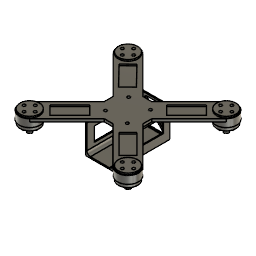
droneframev3 (Autodesk Fusion 360 archive; units mm, degrees)
design "droneTestv2"
part number: 2026-03-09-17-57-18-484
Autodesk Fusion 360 part; units mm, degrees
sketch "Sketch1" plane through (0, 0, 0) normal (0, 0, 1) x (1, 0, 0)
  line L0 (5.1145, 0) -> (50, 0)
  line L1 (55, -5) -> (55, -50)
  line L2 (50, -55) -> (5, -55)
  line L3 (0, -50) -> (0, -5.1145)
  circle A0 centre (12, -11) radius 2
  circle A1 centre (43, -11) radius 2
  circle A2 centre (12, -44) radius 2
  circle A3 centre (43, -44) radius 2
  line L4 (0, -5.1145) -> (0, 0)
  line L5 (0, 0) -> (5.1145, 0)
  line L6 (50, 0) -> (55, 0)
  line L7 (55, 0) -> (55, -5)
  line L8 (50, -55) -> (55, -55)
  line L9 (55, -55) -> (55, -50)
  line L10 (0, -50) -> (0, -55)
  line L11 (0, -55) -> (5, -55)
  line L12 (0, -21.2132) -> (21.2132, 0)
  line L13 (21.2132, 0) -> (-31.8198, 53.033)
  line L14 (-31.8198, 53.033) -> (-53.033, 31.8198)
  line L15 (-53.033, 31.8198) -> (0, -21.2132)
  line L16 (21.2132, -55) -> (0, -33.7868)
  line L17 (0, -33.7868) -> (-53.033, -86.8198)
  line L18 (-53.033, -86.8198) -> (-31.8198, -108.033)
  line L19 (-31.8198, -108.033) -> (21.2132, -55)
  line L20 (33.7868, -55) -> (55, -33.7868)
  line L21 (55, -33.7868) -> (108.033, -86.8198)
  line L22 (108.033, -86.8198) -> (86.8198, -108.033)
  line L23 (86.8198, -108.033) -> (33.7868, -55)
  line L24 (33.7868, 0) -> (55, -21.2132)
  line L25 (55, -21.2132) -> (108.033, 31.8198)
  line L26 (108.033, 31.8198) -> (86.8198, 53.033)
  line L27 (86.8198, 53.033) -> (33.7868, 0)
  circle A4 centre (-40, -95) radius 64.77
  circle A5 centre (95, -95) radius 64.77
  circle A6 centre (-40, 40) radius 64.77
  circle A7 centre (95, 40) radius 64.77
  circle A8 centre (97.4264, -97.4264) radius 8
  circle A9 centre (97.4264, -89.4264) radius 2
  circle A10 centre (105.4264, -97.4264) radius 2
  circle A11 centre (97.4264, -105.4264) radius 2
  circle A12 centre (89.4264, -97.4264) radius 2
  circle A13 centre (97.4264, -97.4264) radius 13.75
  circle A14 centre (97.4264, -97.4264) radius 15
  circle A15 centre (-42.4264, -97.4264) radius 8
  circle A16 centre (-42.4264, -105.4264) radius 2
  circle A17 centre (-50.4264, -97.4264) radius 2
  circle A18 centre (-42.4264, -89.4264) radius 2
  circle A19 centre (-34.4264, -97.4264) radius 2
  circle A20 centre (-42.4264, -97.4264) radius 13.75
  circle A21 centre (-42.4264, -97.4264) radius 15
  circle A22 centre (-42.4264, 42.4264) radius 8
  circle A23 centre (-50.4264, 42.4264) radius 2
  circle A24 centre (-42.4264, 50.4264) radius 2
  circle A25 centre (-34.4264, 42.4264) radius 2
  circle A26 centre (-42.4264, 34.4264) radius 2
  circle A27 centre (-42.4264, 42.4264) radius 15
  circle A28 centre (-42.4264, 42.4264) radius 13.75
  circle A29 centre (97.4264, 42.4264) radius 15
  circle A30 centre (97.4264, 42.4264) radius 13.75
  circle A31 centre (97.4264, 42.4264) radius 8
  circle A32 centre (97.4264, 50.4264) radius 2
  circle A33 centre (105.4264, 42.4264) radius 2
  circle A34 centre (97.4264, 34.4264) radius 2
  circle A35 centre (89.4264, 42.4264) radius 2
  circle A36 centre (97.4264, -105.4264) radius 3
  circle A37 centre (89.4264, -97.4264) radius 3
  circle A38 centre (97.4264, -89.4264) radius 3
  circle A39 centre (105.4264, -97.4264) radius 3
  circle A40 centre (105.4264, 42.4264) radius 3
  circle A41 centre (97.4264, 50.4264) radius 3
  circle A42 centre (89.4264, 42.4264) radius 3
  circle A43 centre (97.4264, 34.4264) radius 3
  circle A44 centre (-34.4264, 42.4264) radius 3
  circle A45 centre (-42.4264, 50.4264) radius 3
  circle A46 centre (-50.4264, 42.4264) radius 3
  circle A47 centre (-42.4264, 34.4264) radius 3
  circle A48 centre (-42.4264, -89.4264) radius 3
  circle A49 centre (-50.4264, -97.4264) radius 3
  circle A50 centre (-34.4264, -97.4264) radius 3
  circle A51 centre (-42.4264, -105.4264) radius 3
  point P0 (55, 0)
  point P1 (0, -55)
  dimension "d1" = 55
  dimension "d2" = 55
  dimension "d7" = 4
  dimension "d8" = 12
  dimension "d9" = 11
  dimension "d11" = 4
  dimension "d12" = 12
  dimension "d13" = 11
  dimension "d14" = 4
  dimension "d15" = 11
  dimension "d16" = 12
  dimension "d17" = 4
  dimension "d18" = 12
  dimension "d19" = 11
  dimension "d22" = 75
  dimension "d23" = 30
  dimension "d24" = 75
  dimension "d25" = 30
  dimension "d26" = 75
  dimension "d27" = 30
  dimension "d28" = 75
  dimension "d29" = 30
  dimension "d31" = 129.54
  dimension "d32" = 129.54
  dimension "d33" = 129.54
  dimension "d34" = 129.54
  dimension "d49" = 16
  dimension "d52" = 4
  dimension "d53" = 4
  dimension "d54" = 4
  dimension "d55" = 4
  dimension "d56" = 27.5
  dimension "d57" = 16
  dimension "d58" = 4
  dimension "d59" = 4
  dimension "d60" = 4
  dimension "d61" = 4
  dimension "d62" = 27.5
  dimension "d63" = 30
  dimension "d64" = 16
  dimension "d65" = 4
  dimension "d66" = 4
  dimension "d67" = 4
  dimension "d68" = 4
  dimension "d69" = 30
  dimension "d70" = 27.5
  dimension "d71" = 30
  dimension "d72" = 27.5
  dimension "d73" = 16
  dimension "d74" = 4
  dimension "d75" = 4
  dimension "d76" = 4
  dimension "d77" = 4
  dimension "d169" = 6
  dimension "d170" = 6
  dimension "d171" = 6
  dimension "d172" = 6
  dimension "d191" = 6
  dimension "d192" = 6
  dimension "d193" = 6
  dimension "d194" = 6
  dimension "d195" = 6
  dimension "d196" = 6
  dimension "d197" = 6
  dimension "d198" = 6
  dimension "d199" = 6
  dimension "d200" = 6
  dimension "d201" = 6
  dimension "d202" = 6
  constraint horizontal L0
  constraint vertical L1
  constraint horizontal L2
  constraint vertical L3
  constraint coincident L4.end L5.start
  constraint coincident L4.end L0
  constraint coincident L4.end L3
  constraint coincident P0 L1
  constraint coincident P0 L0
  constraint coincident P1 L2
  constraint coincident P1 L3
  constraint coincident P0 L6.end
  constraint parallel L2 L8
  constraint coincident P1 L10.end
  constraint perpendicular L12 L13
  constraint parallel L12 L14
  constraint parallel L13 L15
  constraint coincident L0 L12.end
  constraint coincident L3 L12.start
  constraint perpendicular L16 L17
  constraint parallel L16 L18
  constraint parallel L17 L19
  constraint coincident L3 L16.end
  constraint coincident L2 L16.start
  constraint perpendicular L20 L21
  constraint parallel L20 L22
  constraint parallel L21 L23
  constraint coincident L1 L20.end
  constraint coincident L2 L20.start
  constraint perpendicular L24 L25
  constraint parallel L24 L26
  constraint parallel L25 L27
  constraint coincident L1 L24.end
  constraint coincident L0 L24.start
  constraint midpoint L22 A8.centre
  constraint coincident A8 A9.centre
  constraint coincident A8 A10.centre
  constraint coincident A8 A11.centre
  constraint coincident A8 A12.centre
  constraint concentric A8 A13
  constraint concentric A8 A14
  constraint coincident L22.end A14
  constraint midpoint L18 A15.centre
  constraint coincident A15 A16.centre
  constraint coincident A15 A17.centre
  constraint coincident A15 A18.centre
  constraint coincident A15 A19.centre
  constraint concentric A15 A20
  constraint concentric A20 A21
  constraint midpoint L14 A22.centre
  constraint coincident A22 A23.centre
  constraint coincident A22 A24.centre
  constraint coincident A22 A25.centre
  constraint coincident A22 A26.centre
  constraint concentric A22 A27
  constraint concentric A27 A28
  constraint midpoint L26 A29.centre
  constraint concentric A29 A30
  constraint concentric A30 A31
  constraint coincident A31 A32.centre
  constraint coincident A31 A33.centre
  constraint coincident A31 A34.centre
  constraint coincident A31 A35.centre
  constraint concentric A11 A36
  constraint concentric A12 A37
  constraint concentric A9 A38
  constraint concentric A10 A39
  constraint concentric A33 A40
  constraint concentric A32 A41
  constraint concentric A35 A42
  constraint concentric A34 A43
  constraint concentric A25 A44
  constraint concentric A24 A45
  constraint concentric A23 A46
  constraint concentric A26 A47
  constraint concentric A18 A48
  constraint concentric A17 A49
  constraint concentric A19 A50
  constraint concentric A16 A51
  measures "d1" distance of L4.end P0
  measures "d2" distance of L4.end L10.end
  measures "d7" diameter of A0
  measures "d8" distance of L3 A0.centre
  measures "d9" distance of L0 A0.centre
  measures "d11" diameter of A1
  measures "d12" distance of L1 A1.centre
  measures "d13" distance of L0 A1.centre
  measures "d14" diameter of A2
  measures "d15" distance of L2 A2.centre
  measures "d16" distance of L3 A2.centre
  measures "d17" diameter of A3
  measures "d18" distance of L1 A3.centre
  measures "d19" distance of L2 A3.centre
  measures "d22" distance of L12.start L14.end
  measures "d23" distance of L13 L15
  measures "d24" distance of L16.start L18.end
  measures "d25" distance of L17 L19
  measures "d26" distance of L20.start L22.end
  measures "d27" distance of L21 L23
  measures "d28" distance of L24.start L26.end
  measures "d29" distance of L25 L27
  measures "d31" diameter of A4
  measures "d32" diameter of A5
  measures "d33" diameter of A6
  measures "d34" diameter of A7
  measures "d49" diameter of A8
  measures "d52" diameter of A9
  measures "d53" diameter of A10
  measures "d54" diameter of A11
  measures "d55" diameter of A12
  measures "d56" diameter of A13
  measures "d57" diameter of A15
  measures "d58" diameter of A16
  measures "d59" diameter of A17
  measures "d60" diameter of A18
  measures "d61" diameter of A19
  measures "d62" diameter of A20
  measures "d63" diameter of A21
  measures "d64" diameter of A22
  measures "d65" diameter of A23
  measures "d66" diameter of A24
  measures "d67" diameter of A25
  measures "d68" diameter of A26
  measures "d69" diameter of A27
  measures "d70" diameter of A28
  measures "d71" diameter of A29
  measures "d72" diameter of A30
  measures "d73" diameter of A31
  measures "d74" diameter of A32
  measures "d75" diameter of A33
  measures "d76" diameter of A34
  measures "d77" diameter of A35
  measures "d169" diameter of A36
  measures "d170" diameter of A37
  measures "d171" diameter of A38
  measures "d172" diameter of A39
  measures "d191" diameter of A40
  measures "d192" diameter of A41
  measures "d193" diameter of A42
  measures "d194" diameter of A43
  measures "d195" diameter of A44
  measures "d196" diameter of A45
  measures "d197" diameter of A46
  measures "d198" diameter of A47
  measures "d199" diameter of A48
  measures "d200" diameter of A49
  measures "d201" diameter of A50
  measures "d202" diameter of A51
extrude "Extrude1" add sketch "Sketch1" along normal blind 3 contours L0 L3 A0 L12 A6 | L0 L1 L2 L3 A0 A1 A2 A3 L12 L16 L20 L24 | L0 L13 A6 | L0 L27 A7 | L0 L1 A1 L24 A7 | L0 L3 L4 L5 A6 | L0 L3 L4 L5 L13 L15 A6 A27 | L0 L1 L6 L7 L25 L27 A7 A29 | L0 L1 L6 L7 A7 | L3 L15 A6 | L14 A27 A28 | L14 A27 A28 | L1 L25 A7 | L26 A29 A30 | L26 A29 A30 | L14 A22 A28 A44 A47 | L14 A22 A28 A45 A46 | L26 A30 A31 A40 A41 | L26 A30 A31 A42 A43 | L2 L3 A2 L16 A4 | L3 L17 A4 | L14 A22 A44 A47 | L14 A22 A45 A46 | L1 L21 A5 | L1 L2 A3 L20 A5 | L26 A31 A40 A41 | L26 A31 A42 A43 | L2 L3 L10 L11 A4 | L2 L3 L10 L11 L17 L19 A4 A21 | A22 A25 A44 | A22 A25 A44 | A22 A24 A45 | A22 A24 A45 | L1 L2 L8 L9 L21 L23 A5 A14 | L1 L2 L8 L9 A5 | A31 A32 A41 | A31 A32 A41 | A31 A35 A42 | A31 A35 A42 | L2 L19 A4 | L18 A20 A21 | L18 A20 A21 | A22 A23 A46 | A22 A23 A46 | A22 A26 A47 | A22 A26 A47 | L2 L23 A5 | L22 A13 A14 | L22 A13 A14 | A31 A34 A43 | A31 A34 A43 | A31 A33 A40 | A31 A33 A40 | L18 A15 A20 A48 A50 | L18 A15 A20 A49 A51 | L22 A8 A13 A36 A39 | L22 A8 A13 A37 A38 | L18 A15 A48 A50 | L18 A15 A49 A51 | L22 A8 A36 A39 | L22 A8 A37 A38 | A15 A18 A48 | A15 A18 A48 | A15 A17 A49 | A15 A17 A49 | A8 A10 A39 | A8 A10 A39 | A8 A9 A38 | A8 A9 A38 | A15 A16 A51 | A15 A16 A51 | A15 A19 A50 | A15 A19 A50 | A8 A12 A37 | A8 A12 A37 | A8 A11 A36 | A8 A11 A36 makes body 1
extrude "Extrude2" add 1 faces at (-8.062, 10.5564, 3) along direction (0, 0, 1) blind 1 on bodies 1 bodies 1
extrude "Extrude3" cut sketch "Sketch1" along normal blind 10 contours L14 A22 A28 A44 A47 | L14 A22 A28 A45 A46 | L14 A22 A44 A47 | L14 A22 A45 A46 | A22 A25 A44 | A22 A25 A44 | A22 A24 A45 | A22 A24 A45 | A22 A23 A46 | A22 A23 A46 | A22 A26 A47 | A22 A26 A47 bodies 1
extrude "Extrude4" add sketch "Sketch1" along normal blind 10 contours L14 A22 A28 A44 A47 | L14 A22 A28 A45 A46 | L14 A22 A44 A47 | L14 A22 A45 A46 | A22 A25 A44 | A22 A25 A44 | A22 A24 A45 | A22 A24 A45 | A22 A23 A46 | A22 A23 A46 | A22 A26 A47 | A22 A26 A47 bodies 1
extrude "Extrude5" cut sketch "Sketch1" along normal blind 10 contours L26 A30 A31 A40 A41 | L26 A30 A31 A42 A43 | L26 A31 A40 A41 | L26 A31 A42 A43 | A31 A32 A41 | A31 A32 A41 | A31 A35 A42 | A31 A35 A42 | A31 A34 A43 | A31 A34 A43 | A31 A33 A40 | A31 A33 A40 | L18 A15 A20 A48 A50 | L18 A15 A20 A49 A51 | L22 A8 A13 A36 A39 | L22 A8 A13 A37 A38 | L18 A15 A48 A50 | L18 A15 A49 A51 | L22 A8 A36 A39 | L22 A8 A37 A38 | A15 A18 A48 | A15 A18 A48 | A15 A17 A49 | A15 A17 A49 | A8 A10 A39 | A8 A10 A39 | A8 A9 A38 | A8 A9 A38 | A15 A16 A51 | A15 A16 A51 | A15 A19 A50 | A15 A19 A50 | A8 A12 A37 | A8 A12 A37 | A8 A11 A36 | A8 A11 A36 bodies 1
extrude "Extrude6" add sketch "Sketch1" along normal blind 10 contours L26 A30 A31 A40 A41 | L26 A30 A31 A42 A43 | L26 A31 A40 A41 | L26 A31 A42 A43 | A31 A32 A41 | A31 A32 A41 | A31 A35 A42 | A31 A35 A42 | A31 A34 A43 | A31 A34 A43 | A31 A33 A40 | A31 A33 A40 | L18 A15 A20 A48 A50 | L18 A15 A20 A49 A51 | L22 A8 A13 A36 A39 | L22 A8 A13 A37 A38 | L18 A15 A48 A50 | L18 A15 A49 A51 | L22 A8 A36 A39 | L22 A8 A37 A38 | A15 A18 A48 | A15 A18 A48 | A15 A17 A49 | A15 A17 A49 | A8 A10 A39 | A8 A10 A39 | A8 A9 A38 | A8 A9 A38 | A15 A16 A51 | A15 A16 A51 | A15 A19 A50 | A15 A19 A50 | A8 A12 A37 | A8 A12 A37 | A8 A11 A36 | A8 A11 A36 bodies 1
extrude "Extrude7" cut 4 faces at (97.346, 40.4215, 10) (-42.5068, 44.4313, 10) (-42.346, -95.4215, 10) (97.346, -99.4313, 10) along direction (0, 0, -1) blind 5 on bodies 1 bodies 1
extrude "Extrude8" add 1 faces at (97.346, -99.4313, 5) along direction (0, 0, -1) blind 6 on bodies 1 bodies 1
extrude "Extrude9" add 1 faces at (97.346, -99.4313, -1) along direction (0, 0, 1) blind 2 on bodies 1 bodies 1
extrude "Extrude10" add 1 faces at (97.346, -99.4313, -1) along direction (0, 0, -1) blind 2 on bodies 1 bodies 1
extrude "Extrude11" add sketch "Sketch1" against normal blind 7 contours L22 A8 A36 A39 | L22 A8 A37 A38 | A8 A10 A39 | A8 A9 A38 | A8 A12 A37 | A8 A11 A36 | A8 A10 | A8 A9 | A8 A12 | A8 A11 picked at (104.6818, -99.8582) picked at (99.8582, -90.171) picked at (90.1642, -99.8605) picked at (99.8582, -104.6818) picked at (104.7781, -97.839) picked at (96.813, -90.0523) picked at (90.0523, -96.813) picked at (96.813, -104.8005) bodies 1
extrude "Extrude12" add sketch "Sketch1" against normal blind 5 contours A8 A10 | A8 A9 | A8 A12 | A8 A11 picked at (106.0247, -97.9232) picked at (98.0975, -88.8726) picked at (88.8675, -96.764) picked at (98.0975, -105.9803) bodies 1
extrude "Extrude13" add sketch "Sketch1" against normal blind 3 contours L26 A30 A31 A40 A41 | L26 A30 A31 A42 A43 | A31 A32 A41 | A31 A35 A42 | A31 A34 A43 | A31 A33 A40 picked at (94.9952, 50.4291) picked at (89.4207, 44.8573) picked at (94.9952, 34.4237) picked at (105.428, 39.9955) bodies 1
extrude "Extrude14" add sketch "Sketch1" against normal blind 6 contours A31 A32 | A31 A35 | A31 A34 | A31 A33 picked at (98.0975, 50.9803) picked at (88.8675, 41.764) picked at (98.0975, 33.8726) picked at (106.0247, 41.9296) bodies 1
extrude "Extrude15" add sketch "Sketch1" against normal blind 7 contours L26 A31 A40 A41 | L26 A31 A42 A43 | A31 A32 A41 | A31 A35 A42 | A31 A34 A43 | A31 A33 A40 | A31 A32 | A31 A35 | A31 A34 | A31 A33 picked at (94.9947, 49.6818) picked at (90.1642, 39.9923) picked at (94.9947, 35.171) picked at (104.6818, 44.8582) picked at (98.0399, 49.8005) picked at (90.0523, 41.813) picked at (96.813, 35.0523) picked at (104.7781, 42.0138) bodies 1
extrude "Extrude16" add sketch "Sketch1" against normal blind 3 contours L14 A22 A28 A44 A47 | L14 A22 A28 A45 A46 | A22 A25 A44 | A22 A24 A45 | A22 A23 A46 | A22 A26 A47 picked at (-34.4248, 39.9955) picked at (-44.8576, 50.4291) picked at (-50.4321, 44.8573) picked at (-44.8576, 34.4237) bodies 1
extrude "Extrude17" add sketch "Sketch1" against normal blind 6 contours A22 A25 | A22 A24 | A22 A23 | A22 A26 picked at (-33.8281, 41.9296) picked at (-41.7553, 50.9803) picked at (-50.9853, 43.0888) picked at (-41.7553, 33.8726) bodies 1
extrude "Extrude18" add sketch "Sketch1" against normal blind 7 contours L14 A22 A44 A47 | L14 A22 A45 A46 | A22 A25 A44 | A22 A24 A45 | A22 A23 A46 | A22 A26 A47 | A22 A25 | A22 A24 | A22 A23 | A22 A26 picked at (-35.171, 39.9947) picked at (-44.8582, 49.6818) picked at (-49.6886, 44.8605) picked at (-44.8582, 35.171) picked at (-35.0747, 42.0138) picked at (-43.0399, 49.8005) picked at (-49.8005, 41.813) picked at (-43.0399, 35.0523) bodies 1
extrude "Extrude19" add sketch "Sketch1" against normal blind 3 contours L18 A15 A20 A48 A50 | L18 A15 A20 A49 A51 | A15 A18 A48 | A15 A17 A49 | A15 A16 A51 | A15 A19 A50 picked at (-44.8576, -89.4237) picked at (-50.4321, -94.9956) picked at (-44.8576, -105.4291) picked at (-34.4248, -99.8573) bodies 1
extrude "Extrude20" add sketch "Sketch1" against normal blind 6 contours A15 A18 | A15 A17 | A15 A16 | A15 A19 picked at (-41.7553, -88.8726) picked at (-50.9853, -96.764) picked at (-41.7553, -105.9803) picked at (-33.8281, -96.9296) bodies 1
extrude "Extrude21" add sketch "Sketch1" against normal blind 7 contours L18 A15 A48 A50 | L18 A15 A49 A51 | A15 A18 A48 | A15 A17 A49 | A15 A16 A51 | A15 A19 A50 | A15 A18 | A15 A17 | A15 A16 | A15 A19 picked at (-39.9947, -90.171) picked at (-49.6886, -99.8605) picked at (-44.8582, -104.6818) picked at (-35.171, -94.9947) picked at (-43.0399, -90.0523) picked at (-49.8005, -96.813) picked at (-43.0399, -104.8005) picked at (-35.0747, -97.839) bodies 1
extrude "Extrude22" add sketch "Sketch1" against normal blind 12 contours L22 A8 A13 A36 A39 | L22 A8 A13 A37 A38 | A8 A10 A39 | A8 A9 A38 | A8 A12 A37 | A8 A11 A36 picked at (105.428, -99.8573) picked at (94.9952, -89.4237) picked at (89.4207, -94.9956) picked at (94.9952, -105.4291) bodies 1
extrude "Extrude23" add sketch "Sketch1" against normal blind 7 contours L22 A13 A14 | L22 A13 A14 bodies 1
extrude "Extrude24" add sketch "Sketch1" against normal blind 7 contours L22 A13 A14 | L22 A13 A14 bodies 1
extrude "Extrude25" cut sketch "Sketch1" along normal blind -30 and the other way blind -6 contours A8 A10 A39 | A8 A10 A39 | A8 A10 | A8 A10 bodies 1
extrude "Extrude26" add sketch "Sketch1" along normal blind 5 contours A8 A10 A39 | A8 A10 A39 bodies 1
extrude "Extrude27" add 1 faces at (94.1257, -99.2826, -7) along direction (0, 0, -1) blind 11 on bodies 1 bodies 1
extrude "Extrude28" cut sketch "Sketch1" along normal mid plane 60 contours A8 A9 A38 | A8 A9 A38 | A8 A12 A37 | A8 A12 A37 | A8 A11 A36 | A8 A11 A36 | A8 A9 | A8 A9 | A8 A12 | A8 A12 | A8 A11 | A8 A11 bodies 1
extrude "Extrude29" add sketch "Sketch1" along normal blind 5 contours A8 A9 A38 | A8 A9 A38 | A8 A12 A37 | A8 A12 A37 | A8 A11 A36 | A8 A11 A36 bodies 1
extrude "Extrude30" add sketch "Sketch1" against normal blind 7 contours L26 A29 A30 | L26 A29 A30 bodies 1
extrude "Extrude31" add sketch "Sketch1" against normal blind 12 separate body contours L26 A30 A31 A40 A41 | L26 A30 A31 A42 A43 | A31 A32 A41 | A31 A35 A42 | A31 A34 A43 | A31 A33 A40 picked at (94.9952, 50.4291) picked at (89.4207, 44.8573) picked at (94.9952, 34.4237) picked at (105.428, 39.9955) makes body 2
extrude "Extrude32" add sketch "Sketch1" against normal blind 19 separate body contours L26 A31 A40 A41 | L26 A31 A42 A43 | A31 A32 A41 | A31 A35 A42 | A31 A34 A43 | A31 A33 A40 picked at (94.9947, 49.6818) picked at (90.1642, 39.9923) picked at (94.9947, 35.171) picked at (104.6818, 44.8582) makes body 3
extrude "Extrude33" cut sketch "Sketch1" along normal mid plane 40 contours A31 A32 A41 | A31 A32 A41 | A31 A35 A42 | A31 A35 A42 | A31 A34 A43 | A31 A34 A43 | A31 A33 A40 | A31 A33 A40 | A31 A32 | A31 A32 | A31 A35 | A31 A35 | A31 A34 | A31 A34 | A31 A33 | A31 A33 bodies 1 2 3
extrude "Extrude34" add sketch "Sketch1" along normal blind 5 contours A31 A32 A41 | A31 A32 A41 | A31 A35 A42 | A31 A35 A42 | A31 A34 A43 | A31 A34 A43 | A31 A33 A40 | A31 A33 A40 bodies 1 2 3
extrude "Extrude35" add sketch "Sketch1" against normal blind 19 separate body contours L14 A22 A44 A47 | L14 A22 A45 A46 makes body 4
extrude "Extrude36" add sketch "Sketch1" against normal blind 19 separate body contours L14 A22 A28 A44 A47 | L14 A22 A28 A45 A46 makes body 5
extrude "Extrude37" cut 1 faces at (-47.5438, 51.3129, -19) along direction (0, 0, 1) blind 7 on bodies 5 bodies 5
extrude "Extrude38" add sketch "Sketch1" against normal blind 7 contours L14 A27 A28 | L14 A27 A28 bodies 1 5
extrude "Extrude39" cut sketch "Sketch1" along normal mid plane 40 contours A22 A25 A44 | A22 A25 A44 | A22 A24 A45 | A22 A24 A45 | A22 A23 A46 | A22 A23 A46 | A22 A26 A47 | A22 A26 A47 | A22 A25 | A22 A25 | A22 A24 | A22 A24 | A22 A23 | A22 A23 | A22 A26 | A22 A26 bodies 1
extrude "Extrude40" add sketch "Sketch1" along normal blind 5 contours A22 A25 A44 | A22 A25 A44 | A22 A24 A45 | A22 A24 A45 | A22 A23 A46 | A22 A23 A46 | A22 A26 A47 | A22 A26 A47 bodies 1 4
extrude "Extrude41" add 1 faces at (-32.1932, -103.3174, -3) along direction (0, 0, -1) blind 9 on bodies 1 bodies 1
extrude "Extrude42" add sketch "Sketch1" against normal blind 7 contours L18 A20 A21 | L18 A20 A21 bodies 1
extrude "Extrude43" add 1 faces at (-41.6768, -95.0423, -7) along direction (0, 0, -1) blind 12 on bodies 1 bodies 1
extrude "Extrude44" cut sketch "Sketch1" along normal mid plane 40 contours A15 A18 A48 | A15 A18 A48 | A15 A17 A49 | A15 A17 A49 | A15 A16 A51 | A15 A16 A51 | A15 A19 A50 | A15 A19 A50 | A15 A18 | A15 A18 | A15 A17 | A15 A17 | A15 A16 | A15 A16 | A15 A19 | A15 A19 bodies 1
extrude "Extrude45" add sketch "Sketch1" along normal blind 5 contours A15 A18 A48 | A15 A18 A48 | A15 A17 A49 | A15 A17 A49 | A15 A16 A51 | A15 A16 A51 | A15 A19 A50 | A15 A19 A50 bodies 1
extrude "Extrude46" add 1 faces at (97.3766, -99.4283, 5) along direction (0, 0, 1) blind 1 on bodies 1 bodies 1
extrude "Extrude47" add 1 faces at (-42.346, -95.4215, 5) along direction (0, 0, 1) blind 1 on bodies 1 bodies 1
extrude "Extrude48" add 1 faces at (-42.3766, 44.4283, 5) along direction (0, 0, 1) blind 1 on bodies 1 bodies 1
extrude "Extrude49" add 1 faces at (97.4762, 40.4245, 5) along direction (0, 0, 1) blind 1 on bodies 1 bodies 1
sketch "Sketch2" plane through (0, 0, 4) normal (0, 0, 1) x (-1, 0, 0)
  circle A0 centre (-97.4264, -42.4264) radius 13.75
  circle A1 centre (-97.4264, 97.4264) radius 13.75
  circle A2 centre (42.4264, 97.4264) radius 13.75
  circle A3 centre (42.4264, -42.4264) radius 13.75
  circle A4 centre (-12, 11) radius 2
  circle A5 centre (-12, 44) radius 2
  circle A6 centre (-43, 11) radius 2
  circle A7 centre (-43, 44) radius 2
  line L0 (-55, 21.2132) -> (-108.033, -31.8198)
  arc A8 (-108.033, -31.8198) -> (-86.8198, -53.033) centre (-97.4264, -42.4264) ccw
  line L1 (-86.8198, -53.033) -> (-33.7868, 0)
  line L2 (-33.7868, 0) -> (-21.2132, 0)
  line L3 (-21.2132, 0) -> (31.8198, -53.033)
  arc A9 (31.8198, -53.033) -> (53.033, -31.8198) centre (42.4264, -42.4264) ccw
  line L4 (53.033, -31.8198) -> (0, 21.2132)
  line L5 (0, 21.2132) -> (0, 33.7868)
  line L6 (0, 33.7868) -> (53.033, 86.8198)
  arc A10 (53.033, 86.8198) -> (31.8198, 108.033) centre (42.4264, 97.4264) ccw
  line L7 (31.8198, 108.033) -> (-21.2132, 55)
  line L8 (-21.2132, 55) -> (-33.7868, 55)
  line L9 (-33.7868, 55) -> (-86.8198, 108.033)
  arc A11 (-86.8198, 108.033) -> (-108.033, 86.8198) centre (-97.4264, 97.4264) ccw
  line L10 (-108.033, 86.8198) -> (-55, 33.7868)
  line L11 (-55, 33.7868) -> (-55, 21.2132)
  line L12 (39.9463, -18.7331) -> (35.6486, -22.92)
  line L13 (35.6486, -22.92) -> (7.7363, 5.7315)
  line L14 (35.6486, -22.92) -> (22.7555, -35.4805)
  line L15 (22.7555, -35.4805) -> (-5.1568, -6.8291)
  line L16 (-5.1568, -6.8291) -> (7.7363, 5.7315)
  line L17 (34.3962, 76.6084) -> (21.6683, 89.3363)
  line L18 (21.6683, 89.3363) -> (-6.6159, 61.052)
  line L19 (-6.6159, 61.052) -> (6.112, 48.3241)
  line L20 (6.112, 48.3241) -> (34.3962, 76.6084)
  line L21 (-83.2843, -28.2843) -> (-76.9203, -34.6482)
  line L22 (-76.9203, -34.6482) -> (-48.636, -6.364)
  line L23 (-48.636, -6.364) -> (-61.364, 6.364)
  line L24 (-61.364, 6.364) -> (-89.6482, -21.9203)
  line L25 (-89.6482, -21.9203) -> (-83.2843, -28.2843)
  line L26 (-97.4264, 97.4264) -> (-83.2843, 83.2843)
  line L27 (-83.2843, 83.2843) -> (-89.6482, 76.9203)
  line L28 (-89.6482, 76.9203) -> (-61.364, 48.636)
  line L29 (-61.364, 48.636) -> (-48.636, 61.364)
  line L30 (-48.636, 61.364) -> (-76.9203, 89.6482)
  line L31 (-76.9203, 89.6482) -> (-83.2843, 83.2843)
  line L32 (42.4264, 97.4264) -> (28.2843, 83.2843)
  line L33 (42.4264, -42.4264) -> (28.4703, -28.1007)
  dimension "d244" = 6
  dimension "d245" = 40
  dimension "d246" = 18
  dimension "d247" = 40
  dimension "d249" = 18
  dimension "d250" = 40
  dimension "d251" = 18
  dimension "d259" = 20
  dimension "d260" = 9
  dimension "d261" = 40
  dimension "d262" = 18
  dimension "d263" = 40
  dimension "d264" = 20
  dimension "d265" = 9
  dimension "d266" = 40
  dimension "d267" = 18
  dimension "d268" = 40
  dimension "d269" = 20
  dimension "d270" = 20
  constraint coincident L4 L12.start
  constraint perpendicular L12 L13
  constraint perpendicular L13 L14
  constraint perpendicular L14 L15
  constraint perpendicular L6 L17
  constraint perpendicular L17 L18
  constraint perpendicular L18 L19
  constraint perpendicular L21 L22
  constraint perpendicular L22 L23
  constraint perpendicular L23 L24
  constraint coincident A1.centre A11.centre
  constraint perpendicular L26 L27
  constraint perpendicular L27 L28
  constraint perpendicular L28 L29
  constraint perpendicular L29 L30
  constraint coincident A2.centre A10.centre
  constraint perpendicular L19 L32
  constraint coincident A3.centre A9.centre
  constraint perpendicular L16 L33
  measures "d244" distance of L12.start L12.end
  measures "d245" distance of L12.end L13.end
  measures "d246" distance of L12.end L14.end
  measures "d247" distance of L14.end L15.end
  measures "d249" distance of L17.start L17.end
  measures "d250" distance of L17.end L18.end
  measures "d251" distance of L18.end L19.end
  measures "d259" distance of A0.centre L21.start
  measures "d260" distance of L21.start L21.end
  measures "d261" distance of L21.end L22.end
  measures "d262" distance of L22.end L23.end
  measures "d263" distance of L23.end L24.end
  measures "d264" distance of A1.centre L26.end
  measures "d265" distance of L26.end L27.end
  measures "d266" distance of L27.end L28.end
  measures "d267" distance of L28.end L29.end
  measures "d268" distance of L29.end L30.end
  measures "d269" distance of A2.centre L32.end
  measures "d270" distance of A3.centre L33.end
extrude "Extrude50" cut sketch "Sketch2" against normal blind 2 contours L13 L14 L15 L16 | L17 L18 L19 L20 | L21 L22 L23 L24 L25 | L27 L28 L29 L30 L31 bodies 1
sketch "Sketch3" plane through (0, 0, 0) normal (0, 0, 1) x (1, 0, 0)
  line L0 (5, -55) -> (7.4275, -67.7242)
  line L1 (7.4275, -67.7242) -> (47.4275, -67.7242)
  line L2 (47.4275, -67.7242) -> (47.4275, 12.2758)
  line L3 (47.4275, 12.2758) -> (7.4275, 12.2758)
  line L4 (7.4275, 12.2758) -> (7.4275, -67.7242)
  line L5 (0, 0) -> (27.5, 0)
  line L6 (0, 0) -> (7.5, 0)
  dimension "d278" = 40
  dimension "d279" = 80
  dimension "d310" = 27.5
  dimension "d312" = 7.5
  constraint horizontal L1
  constraint vertical L2
  constraint horizontal L3
  constraint vertical L4
  constraint coincident L5.start L6.start
  constraint perpendicular L2 L5
  constraint parallel L5 L6
  measures "d278" distance of L0.end L1.end
  measures "d279" distance of L0.end L3.end
  measures "d310" distance of L5.start L5.end
  measures "d312" distance of L5.start L6.end
extrude "Extrude60" add sketch "Sketch3" against normal blind 42 bodies 1
sketch "Sketch7" plane through (0, -67.7242, 0) normal (0, -1, 0) x (1, 0, 0)
  line L0 (8.489, 0) -> (7.4275, 0)
  line L1 (7.4275, 0) -> (7.4275, -42)
  line L2 (7.4275, -42) -> (47.4275, -42)
  line L3 (47.4275, -42) -> (47.4275, 0)
  line L4 (47.4275, 0) -> (46.511, 0)
  line L5 (46.511, 0) -> (8.489, 0)
  line L6 (7.4275, -42) -> (9.4275, -42)
  line L7 (14.2059, -40) -> (41.2059, -40)
  line L8 (46.2059, -35) -> (46.2059, -1)
  line L9 (45.2059, 0) -> (10.2059, 0)
  line L10 (9.2059, -1) -> (9.2059, -35)
  arc A0 (10.2059, 0) -> (9.2059, -1) centre (10.2059, -1) ccw
  arc A1 (46.2059, -1) -> (45.2059, 0) centre (45.2059, -1) ccw
  arc A2 (9.2059, -35) -> (14.2059, -40) centre (14.2059, -35) ccw
  arc A3 (41.2059, -40) -> (46.2059, -35) centre (41.2059, -35) ccw
  point P0 (9.2059, -40)
  point P1 (46.2059, -40)
  point P2 (9.2059, 0)
  dimension "d317" = 2
  dimension "d318" = 37
  dimension "d319" = 40
  dimension "d359" = 1
  dimension "d360" = 1
  dimension "d361" = 5
  dimension "d362" = 5
  dimension "d363" = 42
  constraint coincident L1.end L2.start
  constraint perpendicular L1 L6
  constraint horizontal L7
  constraint vertical L8
  constraint horizontal L9
  constraint vertical L10
  constraint coincident L5 P2
  constraint coincident P2 L9
  constraint coincident P2 L10
  constraint tangent L9 A0
  constraint tangent L10 A0
  constraint tangent L9 A1
  constraint tangent L8 A1
  constraint coincident P0 L10
  constraint coincident P0 L7
  constraint tangent L10 A2
  constraint tangent L7 A2
  constraint coincident P1 L7
  constraint coincident P1 L8
  constraint tangent L7 A3
  constraint tangent L8 A3
  measures "d317" distance of L1.end L6.end
  measures "d318" distance of P0 P1
  measures "d319" distance of P0 P2
  measures "d359" radius of A0
  measures "d360" radius of A1
  measures "d361" radius of A2
  measures "d362" radius of A3
  measures "d363" distance of L2.end L3.end
extrude "Extrude61" cut sketch "Sketch7" against normal blind 78 contours L5 L7 L8 L9 L10 A0 A1 A2 A3 bodies 1
sketch "Sketch8" plane through (0, 12.2758, 0) normal (0, 1, 0) x (-1, 0, 0)
  line L0 (-46.0626, 0) -> (-47.4275, 0)
  line L1 (-47.4275, 0) -> (-47.4275, -42)
  line L2 (-47.4275, -42) -> (-7.4275, -42)
  line L3 (-7.4275, -42) -> (-7.4275, 0)
  line L4 (-7.4275, 0) -> (-8.9374, 0)
  line L5 (-8.9374, 0) -> (-46.0626, 0)
  line L6 (-47.4275, 0) -> (-42.4275, 0)
  line L7 (-7.4275, 0) -> (-12.4275, 0)
  line L8 (-7.4275, 0) -> (-7.4275, -5)
  line L9 (-7.4275, -42) -> (-7.4275, -37)
  line L10 (-7.4275, -42) -> (-12.4275, -42)
  line L11 (-44.4275, -5) -> (-12.4275, -39)
  line L12 (-42.4275, -3) -> (-10.4275, -37)
  line L13 (-44.4275, -37) -> (-12.4275, -3)
  line L14 (-42.4275, -39) -> (-10.4275, -5)
  line L15 (-42.4275, -3) -> (-44.4275, -3)
  line L16 (-44.4275, -3) -> (-44.4275, -5)
  line L17 (-44.4275, -37) -> (-44.4275, -39)
  line L18 (-44.4275, -39) -> (-42.4275, -39)
  line L19 (-37.4275, -39) -> (-17.4275, -39)
  line L20 (-44.4275, -32) -> (-44.4275, -10)
  line L21 (-17.4275, -3) -> (-37.4275, -3)
  line L22 (-12.4275, -3) -> (-10.4275, -2.9988)
  line L23 (-10.4275, -10) -> (-10.4275, -32)
  line L24 (-12.4275, -39) -> (-18.6546, -39)
  arc A0 (-37.4275, -3) -> (-44.4275, -10) centre (-37.4275, -10) ccw
  arc A1 (-10.4275, -10) -> (-17.4275, -3) centre (-17.4275, -10) ccw
  arc A2 (-44.4275, -32) -> (-37.4275, -39) centre (-37.4275, -32) ccw
  arc A3 (-17.4275, -39) -> (-10.4275, -32) centre (-17.4275, -32) ccw
  dimension "d322" = 5
  dimension "d323" = 3
  dimension "d330" = 5
  dimension "d331" = 3
  dimension "d332" = 5
  dimension "d333" = 3
  dimension "d334" = 5
  dimension "d335" = 3
  dimension "d336" = 5
  dimension "d337" = 3
  dimension "d355" = 7
  dimension "d356" = 7
  dimension "d357" = 7
  constraint coincident L0.end L1.start
  constraint perpendicular L1 L6
  constraint coincident L3.end L4.start
  constraint perpendicular L3 L7
  constraint perpendicular L7 L8
  constraint coincident L2.end L3.start
  constraint perpendicular L2 L9
  constraint perpendicular L9 L10
  constraint perpendicular L23 L24
  constraint coincident L12.start L21
  constraint coincident L11.start L20
  constraint tangent L21 A0
  constraint tangent L20 A0
  constraint coincident L13.end L21
  constraint coincident L22.end L23
  constraint tangent L21 A1
  constraint tangent L23 A1
  constraint coincident L13.start L20
  constraint coincident L14.start L19
  constraint tangent L20 A2
  constraint tangent L19 A2
  constraint coincident L12.end L23
  constraint coincident L11.end L19
  constraint tangent L23 A3
  constraint tangent L19 A3
  measures "d322" distance of L0.end L6.end
  measures "d323" distance of L6.end L12.start
  measures "d330" distance of L3.end L7.end
  measures "d331" distance of L7.end L13.end
  measures "d332" distance of L3.end L8.end
  measures "d333" distance of L8.end L14.end
  measures "d334" distance of L2.end L9.end
  measures "d335" distance of L9.end L12.end
  measures "d336" distance of L2.end L10.end
  measures "d337" distance of L10.end L11.end
  measures "d355" radius of A0
  measures "d356" radius of A1
  measures "d357" radius of A2
extrude "Extrude65" cut sketch "Sketch8" against normal blind 2 contours L11 L13 L20 A0 A2 | L12 L13 L21 A0 A1 | L11 L14 L19 L24 A2 A3 | L12 L14 L23 A1 A3 bodies 1
sketch "Sketch9" plane through (47.4275, 0, 0) normal (1, 0, 0) x (0, 1, 0)
  line L0 (12.2758, 0) -> (-67.7242, 0)
  line L1 (-67.7242, 0) -> (-67.7242, -42)
  line L2 (-67.7242, -42) -> (12.2758, -42)
  line L3 (12.2758, -42) -> (12.2758, 0)
  line L4 (-67.7242, 0) -> (-57.7242, 0)
  line L5 (-57, -10) -> (3, -10)
  line L6 (3, -10) -> (3, -30)
  line L7 (3, -30) -> (-57, -30)
  line L8 (-57, -30) -> (-57, -10)
  line L9 (-57, -10) -> (-29, -10)
  line L10 (-29, -10) -> (-26, -10)
  line L11 (-26, -10) -> (-26, -30)
  line L12 (-26, -30) -> (-29, -30)
  line L13 (-29, -30) -> (-29, -10)
  dimension "d346" = 10
  dimension "d348" = 60
  dimension "d349" = 20
  dimension "d350" = 28
  dimension "d351" = 3
  dimension "d352" = 20
  constraint coincident L0.end L1.start
  constraint perpendicular L1 L4
  constraint horizontal L5
  constraint vertical L6
  constraint horizontal L7
  constraint vertical L8
  constraint perpendicular L8 L9
  constraint horizontal L10
  constraint vertical L11
  constraint horizontal L12
  constraint vertical L13
  measures "d346" distance of L0.end L4.end
  measures "d348" distance of L5.start L5.end
  measures "d349" distance of L5.start L7.end
  measures "d350" distance of L5.start L9.end
  measures "d351" distance of L9.end L10.end
  measures "d352" distance of L9.end L12.end
extrude "Extrude66" cut sketch "Sketch9" against normal blind 42 contours L5 L7 L8 L9 L13 | L5 L6 L7 L11 bodies 1
